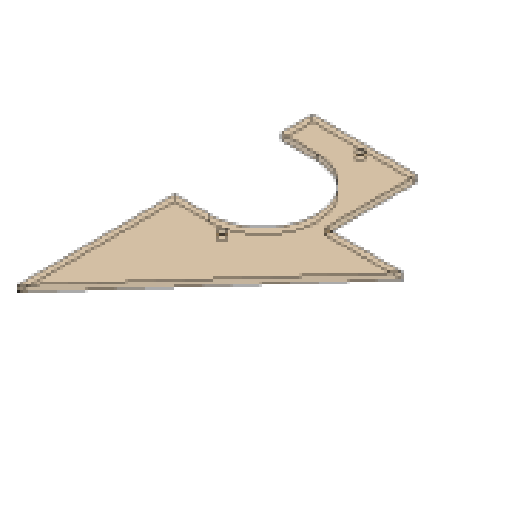
# Autodesk Inventor part: FoldedGuides
Saved by Autodesk Inventor 2023 (Build 270158000, 158)
## iProperties
Created: 2022-11-11
Part Number: FoldedGuides
Material: Polycarbonate, Smoke
Document SubType Name: Modeling
Designer: deli
Density: 1.2 g/cm^3
Appearance: Polycarbonate - Smoked
Author: deli
Autodesk Inventor part; units mm, degrees
ref_plane "YZ Plane" through (0, 0, 0) normal (1, 0, 0) x (0, 1, 0)
ref_plane "XZ Plane" through (0, 0, 0) normal (0, 1, 0) x (-1, 0, 0)
ref_plane "XY Plane" through (0, 0, 0) normal (0, 0, 1) x (1, 0, 0)
sketch "Sketch1" plane through (0, 0, 0) normal (0, 1, 0) x (-1, 0, 0)
  line L0 (-38.0759, 100.3361) -> (-38.0759, 84.3361)
  line L1 (-130.0759, -17.0635) -> (-68.2654, 100.3361)
  circle A0 centre (-130.2509, 71.1844) radius 41.267 construction
  line L2 (-68.2654, 100.3361) -> (-38.0759, 100.3361)
  line L3 (-68.2654, 100.3361) -> (-38.0759, 157.6767)
  line L4 (-38.0759, 157.6767) -> (-38.0759, 100.3361)
  line L5 (-55.9009, 30.4361) -> (-38.0759, 30.4361)
  line L6 (-38.0759, 30.4361) -> (-38.0759, 14.4361)
  line L7 (-38.0759, 14.4361) -> (-92.8509, 14.4361)
  line L8 (-92.8509, 14.4361) -> (-92.8509, -17.0635)
  line L9 (-55.9009, 84.3361) -> (-38.0759, 84.3361)
  line L10 (-92.8509, -17.0635) -> (-130.0759, -17.0635)
  arc A1 (-55.9009, 84.3361) -> (-55.9009, 30.4361) centre (-55.9009, 57.3861) ccw
  circle A2 centre (-66.0759, 18.4361) radius 1.939
  circle A3 centre (-66.0759, 88.4361) radius 2
  line L11 (-61.8868, 112.4513) -> (-38.0759, 112.4513)
  point P0 (0, 0)
  dimension "d4" = 82.534
  dimension "d6" = 92.175
  dimension "d12" = 16
  dimension "d13" = 92
  dimension "d15" = 16
  dimension "d16" = 85.9
  dimension "d17" = 17.825
  dimension "d18" = 4
  dimension "d20" = 4
  dimension "d21" = 28
  dimension "d22" = 28
  dimension "d23" = 10
  dimension "d24" = 29.1518
  dimension "d25" = 4
  dimension "d26" = 41.267
  dimension "d27" = 70
  constraints: 24 end point, 6 perpendicular, 4 centre point, 3 collinear, 3 tangent, 2 point on circle, 2 point on line, 1 horizontal, 1 vertical
  measures "d4" diameter of A0
  measures "d6" distance from line of L0 A0.centre
  measures "d12" distance between parallel lines of L5 L7
  measures "d13" distance from line of L1.start L0
  measures "d15" distance between parallel lines of L2 L9
  measures "d16" distance between parallel lines of L2 L7
  measures "d17" distance from line of A1.centre L0
  measures "d18" diameter of A3
  measures "d20" distance from line of L7 A2.centre
  measures "d21" distance from line of L6 A2.centre
  measures "d22" distance from line of L0 A3.centre
  measures "d23" distance edge to line of A1 L8
  measures "d24" distance from line of A0.centre L2
  measures "d25" distance edge to line of A1 L1
  measures "d26" distance from line of A0.centre L11
  measures "d27" distance of A2.centre A3.centre
extrude "Extrusion1" add sketch "Sketch1" along normal blind 3.175 contours L0 L9 A1 L5 L6 L7 L8 L10 L1 L2
equation "\"d15\" = d12"
equation "\"d22\" = d21"
equation "\"d26\" = 0.5 * d4"
body "Solid1"
